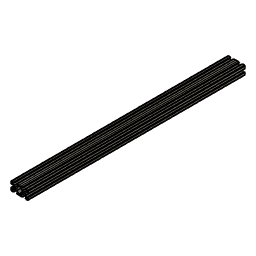
2040-extrusion (Autodesk Fusion 360 design; units mm, degrees)
Autodesk Fusion 360 part; units mm, degrees
sketch "Sketch1" plane through (0, 0, 0) normal (0, 1, 0) x (1, 0, 0)
  line L0 (9, -10) -> (-9, -10)
  line L1 (-10, -9) -> (-10, 9)
  line L2 (-9, 10) -> (9, 10)
  line L3 (10, 9) -> (10, -9)
  line L4 (10, -10) -> (-10, 10) construction
  line L5 (-10, -10) -> (10, 10) construction
  line L6 (4, -4) -> (-4, -4)
  line L7 (-4, -4) -> (-4, 4)
  line L8 (-4, 4) -> (4, 4)
  line L9 (4, 4) -> (4, -4)
  line L10 (4, -4) -> (-4, 4) construction
  line L11 (-4, -4) -> (4, 4) construction
  circle A0 centre (0, 0) radius 2
  line L12 (8.45, -8.45) -> (-8.45, -8.45)
  line L13 (-8.45, -8.45) -> (-8.45, 8.45)
  line L14 (-8.45, 8.45) -> (8.45, 8.45)
  line L15 (8.45, 8.45) -> (8.45, -8.45)
  line L16 (8.45, -8.45) -> (-8.45, 8.45) construction
  line L17 (-8.45, -8.45) -> (8.45, 8.45) construction
  line L18 (-9.452, -10.548) -> (10.548, 9.452) construction
  line L19 (-10.548, -9.452) -> (9.452, 10.548) construction
  line L20 (10.548, -9.452) -> (-9.452, 10.548) construction
  line L21 (9.452, -10.548) -> (-10.548, 9.452) construction
  line L22 (3.1, -10) -> (-3.1, -10) construction
  line L23 (-3.1, -10) -> (-3.1, 10) construction
  line L24 (-3.1, 10) -> (3.1, 10) construction
  line L25 (3.1, 10) -> (3.1, -10) construction
  line L26 (10, -3.1) -> (-10, -3.1) construction
  line L27 (-10, -3.1) -> (-10, 3.1) construction
  line L28 (-10, 3.1) -> (10, 3.1) construction
  line L29 (10, 3.1) -> (10, -3.1) construction
  line L30 (-3.1, -8.45) -> (-3.1, -10)
  line L31 (3.1, -8.45) -> (3.1, -10)
  line L32 (-8.45, -3.1) -> (-10, -3.1)
  line L33 (-8.45, 3.1) -> (-10, 3.1)
  line L34 (8.45, -3.1) -> (10, -3.1)
  line L35 (8.45, 3.1) -> (10, 3.1)
  line L36 (-3.1, 8.45) -> (-3.1, 10)
  line L37 (3.1, 8.45) -> (3.1, 10)
  line L38 (-4, 2.904) -> (-8.45, 7.354)
  line L39 (-2.904, 4) -> (-7.354, 8.45)
  line L40 (2.904, 4) -> (7.354, 8.45)
  line L41 (4, 2.904) -> (8.45, 7.354)
  line L42 (-4, -2.904) -> (-8.45, -7.354)
  line L43 (-2.904, -4) -> (-7.354, -8.45)
  line L44 (2.904, -4) -> (7.354, -8.45)
  line L45 (4, -2.904) -> (8.45, -7.354)
  line L46 (-10, -3.1) -> (-9.55, -3.1)
  line L47 (-9.55, -3.1) -> (-9.55, -3.6)
  line L48 (-9.55, -3.6) -> (-10, -3.6)
  line L49 (-10, -3.6) -> (-10, -3.1)
  line L50 (-10, 3.1) -> (-9.55, 3.1)
  line L51 (-9.55, 3.1) -> (-9.55, 3.6)
  line L52 (-9.55, 3.6) -> (-10, 3.6)
  line L53 (-10, 3.6) -> (-10, 3.1)
  line L54 (-3.1, -10) -> (-3.6, -10)
  line L55 (-3.6, -10) -> (-3.6, -9.55)
  line L56 (-3.6, -9.55) -> (-3.1, -9.55)
  line L57 (-3.1, -9.55) -> (-3.1, -10)
  line L58 (3.1, -10) -> (3.6, -10)
  line L59 (3.6, -10) -> (3.6, -9.55)
  line L60 (3.6, -9.55) -> (3.1, -9.55)
  line L61 (3.1, -9.55) -> (3.1, -10)
  line L62 (10, -3.1) -> (9.55, -3.1)
  line L63 (9.55, -3.1) -> (9.55, -3.6)
  line L64 (9.55, -3.6) -> (10, -3.6)
  line L65 (10, -3.6) -> (10, -3.1)
  line L66 (10, 3.1) -> (9.55, 3.1)
  line L67 (9.55, 3.1) -> (9.55, 3.6)
  line L68 (9.55, 3.6) -> (10, 3.6)
  line L69 (10, 3.6) -> (10, 3.1)
  line L70 (-3.1, 10) -> (-3.6, 10)
  line L71 (-3.6, 10) -> (-3.6, 9.55)
  line L72 (-3.6, 9.55) -> (-3.1, 9.55)
  line L73 (-3.1, 9.55) -> (-3.1, 10)
  line L74 (3.1, 10) -> (3.55, 10)
  line L75 (3.55, 10) -> (3.55, 9.5)
  line L76 (3.55, 9.5) -> (3.1, 9.5)
  line L77 (3.1, 9.5) -> (3.1, 10)
  arc A1 (-10, -9) -> (-9, -10) centre (-9, -9) ccw
  arc A2 (9, -10) -> (10, -9) centre (9, -9) ccw
  arc A3 (10, 9) -> (9, 10) centre (9, 9) ccw
  arc A4 (-9, 10) -> (-10, 9) centre (-9, 9) ccw
  arc A5 (29, -10) -> (30, -9) centre (29, -9) ccw
  line L78 (30, -3.1) -> (10, -3.1) construction
  line L79 (30, 9) -> (30, -9)
  line L80 (24, 4) -> (24, -4)
  line L81 (29.452, -10.548) -> (9.452, 9.452) construction
  line L82 (30, 3.1) -> (29.55, 3.1)
  line L83 (29, -10) -> (11, -10)
  line L84 (16, 4) -> (24, 4)
  line L85 (24, -4) -> (16, 4) construction
  line L86 (28.45, -8.45) -> (11.55, -8.45)
  circle A6 centre (20, 0) radius 2
  line L87 (10, -9) -> (10, 9)
  line L88 (10, -3.1) -> (10, 3.1) construction
  line L89 (16.9, 8.45) -> (16.9, 10)
  arc A7 (11, 10) -> (10, 9) centre (11, 9) ccw
  line L90 (17.096, -4) -> (12.646, -8.45)
  line L91 (16.9, -8.45) -> (16.9, -10)
  line L92 (16.4, -9.55) -> (16.9, -9.55)
  line L93 (10, -3.1) -> (10.45, -3.1)
  line L94 (10, 3.1) -> (10.45, 3.1)
  line L95 (10.45, 3.1) -> (10.45, 3.6)
  arc A8 (10, -9) -> (11, -10) centre (11, -9) ccw
  line L96 (10.45, -3.1) -> (10.45, -3.6)
  line L97 (16.9, -10) -> (16.9, 10) construction
  line L98 (10.45, -3.6) -> (10, -3.6)
  line L99 (29.55, 3.1) -> (29.55, 3.6)
  line L100 (16, -4) -> (16, 4)
  line L101 (23.1, -9.55) -> (23.1, -10)
  line L102 (28.45, -3.1) -> (30, -3.1)
  line L103 (30, -3.6) -> (30, -3.1)
  line L104 (22.904, -4) -> (27.354, -8.45)
  line L105 (22.904, 4) -> (27.354, 8.45)
  line L106 (23.1, 10) -> (23.1, -10) construction
  line L107 (16, -2.904) -> (11.55, -7.354)
  line L108 (16, 2.904) -> (11.55, 7.354)
  line L109 (16.4, 10) -> (16.4, 9.55)
  line L110 (17.096, 4) -> (12.646, 8.45)
  line L111 (10, -3.6) -> (10, -3.1)
  line L112 (16.9, -9.55) -> (16.9, -10)
  line L113 (23.1, 9.5) -> (23.1, 10)
  line L114 (23.6, -10) -> (23.6, -9.55)
  line L115 (10.45, 3.6) -> (10, 3.6)
  line L116 (24, -2.904) -> (28.45, -7.354)
  line L117 (23.55, 10) -> (23.55, 9.5)
  line L118 (10, 3.6) -> (10, 3.1)
  line L119 (11.55, 3.1) -> (10, 3.1)
  line L120 (11.55, -8.45) -> (11.55, 8.45)
  line L121 (23.1, -10) -> (23.6, -10)
  line L122 (11.55, -3.1) -> (10, -3.1)
  line L123 (29.55, -3.6) -> (30, -3.6)
  line L124 (16.4, 9.55) -> (16.9, 9.55)
  line L125 (23.1, 10) -> (23.55, 10)
  line L126 (16.9, 10) -> (16.4, 10)
  line L127 (16.4, -10) -> (16.4, -9.55)
  line L128 (10, 3.1) -> (30, 3.1) construction
  line L129 (24, 2.904) -> (28.45, 7.354)
  line L130 (23.55, 9.5) -> (23.1, 9.5)
  line L131 (23.1, -8.45) -> (23.1, -10)
  line L132 (16.9, 9.55) -> (16.9, 10)
  line L133 (23.1, -10) -> (16.9, -10) construction
  line L134 (30, -3.1) -> (29.55, -3.1)
  line L135 (30.548, -9.452) -> (10.548, 10.548) construction
  line L136 (23.6, -9.55) -> (23.1, -9.55)
  line L137 (29.55, -3.1) -> (29.55, -3.6)
  line L138 (16.9, 10) -> (23.1, 10) construction
  line L139 (30, 3.1) -> (30, -3.1) construction
  line L140 (23.1, 8.45) -> (23.1, 10)
  line L141 (16.9, -10) -> (16.4, -10)
  line L142 (24, -4) -> (16, -4)
  line L143 (16, -4) -> (24, 4) construction
  line L144 (10, -10) -> (30, 10) construction
  arc A9 (30, 9) -> (29, 10) centre (29, 9) ccw
  line L145 (11, 10) -> (29, 10)
  line L146 (28.45, 8.45) -> (28.45, -8.45)
  line L147 (9.452, -9.452) -> (29.452, 10.548) construction
  line L148 (30, 3.6) -> (30, 3.1)
  line L149 (28.45, 3.1) -> (30, 3.1)
  line L150 (11.55, -8.45) -> (28.45, 8.45) construction
  line L151 (11.55, 8.45) -> (28.45, 8.45)
  line L152 (29.55, 3.6) -> (30, 3.6)
  line L153 (30, -10) -> (10, 10) construction
  line L154 (28.45, -8.45) -> (11.55, 8.45) construction
  line L155 (10.548, -10.548) -> (30.548, 9.452) construction
  line L156 (9, -10) -> (11, -10)
  line L157 (9, 10) -> (11, 10)
  line L158 (8.45, -8.45) -> (11.55, -8.45)
  line L159 (8.45, 8.45) -> (11.55, 8.45)
  point P0 (20, 0)
  point P1 (20, 0)
  point P2 (20, 0)
  point P3 (20, 0)
  point P4 (20, 0)
  point P5 (20, 0)
  dimension "d1" = 20
  dimension "d2" = 20
  dimension "d3" = 8
  dimension "d4" = 8
  dimension "d5" = 4
  dimension "d6" = 16.9
  dimension "d7" = 16.9
  dimension "d8" = 0.775
  dimension "d9" = -0.775
  dimension "d10" = 0.775
  dimension "d11" = -0.775
  dimension "d12" = 6.2
  dimension "d13" = 20
  dimension "d14" = 20
  dimension "d15" = 6.2
  dimension "d16" = 1.55
  dimension "d17" = 1.55
  dimension "d18" = 1.55
  dimension "d19" = 1.55
  dimension "d20" = 1.55
  dimension "d21" = 1.55
  dimension "d22" = 1.55
  dimension "d23" = 1.55
  dimension "d24" = 0.45
  dimension "d25" = 0.5
  dimension "d26" = 0.45
  dimension "d27" = 0.5
  dimension "d28" = 0.5
  dimension "d29" = 0.45
  dimension "d30" = 0.5
  dimension "d31" = 0.45
  dimension "d32" = 0.45
  dimension "d33" = 0.5
  dimension "d34" = 0.45
  dimension "d35" = 0.5
  dimension "d36" = 0.5
  dimension "d37" = 0.45
  dimension "d38" = 0.45
  dimension "d39" = 0.5
  dimension "d40" = 1
  dimension "d41" = 1
  dimension "d42" = 1
  dimension "d43" = 1
  dimension "d48" = 0.775
  dimension "d49" = -0.775
  dimension "d50" = 0.775
  dimension "d51" = -0.775
  dimension "d52" = 20
  dimension "d53" = 20
  dimension "d54" = 8
  dimension "d55" = 8
  dimension "d56" = 4
  dimension "d57" = 16.9
  dimension "d58" = 16.9
  dimension "d59" = 6.2
  dimension "d60" = 20
  dimension "d61" = 20
  dimension "d62" = 6.2
  dimension "d63" = 1.55
  dimension "d64" = 1.55
  dimension "d65" = 1.55
  dimension "d66" = 1.55
  dimension "d67" = 1.55
  dimension "d68" = 1.55
  dimension "d69" = 1.55
  dimension "d70" = 1.55
  dimension "d71" = 0.45
  dimension "d72" = 0.5
  dimension "d73" = 0.45
  dimension "d74" = 0.5
  dimension "d75" = 0.5
  dimension "d76" = 0.45
  dimension "d77" = 0.5
  dimension "d78" = 0.45
  dimension "d79" = 0.45
  dimension "d80" = 0.5
  dimension "d81" = 0.45
  dimension "d82" = 0.5
  dimension "d83" = 0.5
  dimension "d84" = 0.45
  dimension "d85" = 0.45
  dimension "d86" = 0.5
  dimension "d87" = 1
  dimension "d88" = 1
  dimension "d89" = 1
  dimension "d90" = 1
  constraint horizontal L0
  constraint perpendicular L0 L1
  constraint parallel L0 L2
  constraint parallel L1 L3
  constraint coincident L4 A0.centre
  constraint coincident L5 A0.centre
  constraint coincident A0.centre origin
  constraint horizontal L6
  constraint perpendicular L6 L7
  constraint parallel L6 L8
  constraint parallel L7 L9
  constraint coincident L10 A0.centre
  constraint coincident L11 A0.centre
  constraint horizontal L12
  constraint perpendicular L12 L13
  constraint parallel L12 L14
  constraint parallel L13 L15
  constraint coincident L16 A0.centre
  constraint coincident L17 A0.centre
  constraint horizontal L22
  constraint perpendicular L22 L23
  constraint parallel L22 L24
  constraint parallel L23 L25
  constraint horizontal L26
  constraint perpendicular L26 L27
  constraint parallel L26 L28
  constraint parallel L27 L29
  constraint vertical L30
  constraint coincident L23 L30.start
  constraint coincident L12 L30.start
  constraint vertical L31
  constraint coincident L12 L31.start
  constraint coincident L25 L31.start
  constraint horizontal L32
  constraint coincident L13 L32.start
  constraint coincident L26 L32.start
  constraint horizontal L33
  constraint coincident L13 L33.start
  constraint coincident L28 L33.start
  constraint horizontal L34
  constraint coincident L15 L34.start
  constraint coincident L26 L34.start
  constraint coincident L28 L35.start
  constraint coincident L15 L35.start
  constraint perpendicular L3 L35
  constraint vertical L36
  constraint coincident L14 L36.start
  constraint coincident L23 L36.start
  constraint vertical L37
  constraint coincident L14 L37.start
  constraint coincident L25 L37.start
  constraint coincident L21 L38.start
  constraint coincident L7 L38.start
  constraint coincident L21 L38.end
  constraint coincident L13 L38.end
  constraint coincident L8 L39.start
  constraint coincident L20 L39.start
  constraint coincident L14 L39.end
  constraint coincident L20 L39.end
  constraint coincident L8 L40.start
  constraint coincident L19 L40.start
  constraint coincident L19 L40.end
  constraint coincident L14 L40.end
  constraint coincident L18 L41.start
  constraint coincident L9 L41.start
  constraint coincident L18 L41.end
  constraint coincident L15 L41.end
  constraint coincident L7 L42.start
  constraint coincident L19 L42.start
  constraint coincident L19 L42.end
  constraint coincident L13 L42.end
  constraint coincident L18 L43.start
  constraint coincident L6 L43.start
  constraint coincident L18 L43.end
  constraint coincident L12 L43.end
  constraint coincident L6 L44.start
  constraint coincident L21 L44.start
  constraint coincident L12 L44.end
  constraint coincident L21 L44.end
  constraint coincident L9 L45.start
  constraint coincident L20 L45.start
  constraint coincident L20 L45.end
  constraint coincident L15 L45.end
  constraint horizontal L46
  constraint vertical L47
  constraint horizontal L48
  constraint vertical L49
  constraint horizontal L50
  constraint vertical L51
  constraint horizontal L52
  constraint vertical L53
  constraint horizontal L54
  constraint vertical L55
  constraint horizontal L56
  constraint vertical L57
  constraint horizontal L58
  constraint vertical L59
  constraint horizontal L60
  constraint vertical L61
  constraint horizontal L62
  constraint vertical L63
  constraint horizontal L64
  constraint vertical L65
  constraint horizontal L66
  constraint vertical L67
  constraint horizontal L68
  constraint vertical L69
  constraint horizontal L70
  constraint vertical L71
  constraint horizontal L72
  constraint vertical L73
  constraint horizontal L74
  constraint vertical L75
  constraint horizontal L76
  constraint vertical L77
  constraint coincident L5.start L0
  constraint coincident L5.start L1
  constraint tangent L0 A1
  constraint tangent L1 A1
  constraint coincident L4.start L0
  constraint coincident L4.start L3
  constraint tangent L0 A2
  constraint tangent L3 A2
  constraint coincident L5.end L3
  constraint coincident L5.end L2
  constraint tangent L3 A3
  constraint tangent L2 A3
  constraint coincident L4.end L2
  constraint coincident L4.end L1
  constraint tangent L2 A4
  constraint tangent L1 A4
  constraint horizontal L83
  constraint perpendicular L83 L87
  constraint parallel L83 L145
  constraint parallel L79 L87
  constraint coincident P5 L153
  constraint coincident P5 L144
  constraint coincident P5 P4
  constraint horizontal L142
  constraint perpendicular L100 L142
  constraint parallel L84 L142
  constraint parallel L80 L100
  constraint coincident P5 L85
  constraint coincident P5 L143
  constraint horizontal L86
  constraint perpendicular L86 L120
  constraint parallel L86 L151
  constraint parallel L120 L146
  constraint coincident P5 L154
  constraint coincident P5 L150
  constraint horizontal L133
  constraint perpendicular L97 L133
  constraint parallel L133 L138
  constraint parallel L97 L106
  constraint horizontal L78
  constraint perpendicular L78 L88
  constraint parallel L78 L128
  constraint parallel L88 L139
  constraint vertical L91
  constraint coincident L91.start L97
  constraint coincident L91.start L86
  constraint vertical L131
  constraint coincident L131.start L86
  constraint coincident L131.start L106
  constraint horizontal L122
  constraint coincident L122.start L120
  constraint coincident L122.start L78
  constraint horizontal L119
  constraint coincident L119.start L120
  constraint coincident L119.start L128
  constraint horizontal L102
  constraint coincident L102.start L146
  constraint coincident L102.start L78
  constraint coincident L149.start L128
  constraint coincident L149.start L146
  constraint perpendicular L79 L149
  constraint vertical L89
  constraint coincident L89.start L151
  constraint coincident L89.start L97
  constraint vertical L140
  constraint coincident L140.start L151
  constraint coincident L140.start L106
  constraint coincident L108.start L81
  constraint coincident L108.start L100
  constraint coincident L108.end L81
  constraint coincident L108.end L120
  constraint coincident L110.start L84
  constraint coincident L110.start L135
  constraint coincident L110.end L151
  constraint coincident L110.end L135
  constraint coincident L105.start L84
  constraint coincident L105.start L147
  constraint coincident L105.end L147
  constraint coincident L105.end L151
  constraint coincident L129.start L155
  constraint coincident L129.start L80
  constraint coincident L129.end L155
  constraint coincident L129.end L146
  constraint coincident L107.start L100
  constraint coincident L107.start L147
  constraint coincident L107.end L147
  constraint coincident L107.end L120
  constraint coincident L90.start L155
  constraint coincident L90.start L142
  constraint coincident L90.end L155
  constraint coincident L90.end L86
  constraint coincident L104.start L142
  constraint coincident L104.start L81
  constraint coincident L104.end L86
  constraint coincident L104.end L81
  constraint coincident L116.start L80
  constraint coincident L116.start L135
  constraint coincident L116.end L135
  constraint coincident L116.end L146
  constraint horizontal L93
  constraint vertical L96
  constraint horizontal L98
  constraint vertical L111
  constraint horizontal L94
  constraint vertical L95
  constraint horizontal L115
  constraint vertical L118
  constraint horizontal L141
  constraint vertical L127
  constraint horizontal L92
  constraint vertical L112
  constraint horizontal L121
  constraint vertical L114
  constraint horizontal L136
  constraint vertical L101
  constraint horizontal L134
  constraint vertical L137
  constraint horizontal L123
  constraint vertical L103
  constraint horizontal L82
  constraint vertical L99
  constraint horizontal L152
  constraint vertical L148
  constraint horizontal L126
  constraint vertical L109
  constraint horizontal L124
  constraint vertical L132
  constraint horizontal L125
  constraint vertical L117
  constraint horizontal L130
  constraint vertical L113
  constraint coincident L4.start L83
  constraint coincident L4.start L87
  constraint tangent L83 A8
  constraint tangent L87 A8
  constraint coincident L153.start L83
  constraint coincident L153.start L79
  constraint tangent A5 L83
  constraint tangent A5 L79
  constraint coincident L144.end L79
  constraint coincident L144.end L145
  constraint tangent L79 A9
  constraint tangent A9 L145
  constraint coincident L5.end L145
  constraint coincident L5.end L87
  constraint tangent A7 L145
  constraint tangent L87 A7
  constraint tangent A8 L156
  measures "d1" distance of L4.end L5.end
  measures "d2" distance of L5.start L4.end
  measures "d3" distance of L7.end L8.end
  measures "d4" distance of L6.end L7.end
  measures "d5" diameter of A0
  measures "d6" distance of L13.end L14.end
  measures "d7" distance of L12.end L13.end
  measures "d12" distance of L23.end L24.end
  measures "d13" distance of L22.end L23.end
  measures "d14" distance of L27.end L28.end
  measures "d15" distance of L26.end L27.end
  measures "d16" distance of L30.start L22.end
  measures "d17" distance of L31.start L22.start
  measures "d18" distance of L32.start L26.end
  measures "d19" distance of L33.start L27.end
  measures "d20" distance of L34.start L26.start
  measures "d21" distance of L35.start L28.end
  measures "d22" distance of L36.start L23.end
  measures "d23" distance of L37.start L24.end
  measures "d24" distance of L26.end L46.end
  measures "d25" distance of L26.end L48.end
  measures "d26" distance of L27.end L50.end
  measures "d27" distance of L27.end L52.end
  measures "d28" distance of L22.end L54.end
  measures "d29" distance of L22.end L56.end
  measures "d30" distance of L22.start L58.end
  measures "d31" distance of L22.start L60.end
  measures "d32" distance of L26.start L62.end
  measures "d33" distance of L26.start L64.end
  measures "d34" distance of L28.end L66.end
  measures "d35" distance of L28.end L68.end
  measures "d36" distance of L23.end L70.end
  measures "d37" distance of L23.end L72.end
  measures "d38" distance of L24.end L74.end
  measures "d39" distance of L24.end L76.end
  measures "d40" radius of A1
  measures "d41" radius of A2
  measures "d42" radius of A3
  measures "d43" radius of A4
  measures "d52" distance of L5.end L144.end
  measures "d53" distance of L4.start L5.end
  measures "d54" distance of L80.start L84.start
  measures "d55" distance of L84.start L100.start
  measures "d56" diameter of A6
  measures "d57" distance of L120.end L146.start
  measures "d58" distance of L120.end L86.end
  measures "d59" distance of L89.end L106.start
  measures "d60" distance of L91.end L89.end
  measures "d61" distance of L82.start L28.end
  measures "d62" distance of L26.start L28.end
  measures "d63" distance of L91.start L91.end
  measures "d64" distance of L101.end L131.start
  measures "d65" distance of L26.start L122.start
  measures "d66" distance of L119.start L28.end
  measures "d67" distance of L102.start L78.start
  measures "d68" distance of L149.start L82.start
  measures "d69" distance of L89.start L89.end
  measures "d70" distance of L140.start L106.start
  measures "d71" distance of L26.start L93.end
  measures "d72" distance of L26.start L64.end
  measures "d73" distance of L94.end L28.end
  measures "d74" distance of L68.end L28.end
  measures "d75" distance of L127.start L91.end
  measures "d76" distance of L92.end L91.end
  measures "d77" distance of L101.end L114.start
  measures "d78" distance of L101.end L101.start
  measures "d79" distance of L134.end L78.start
  measures "d80" distance of L103.start L78.start
  measures "d81" distance of L82.end L82.start
  measures "d82" distance of L148.start L82.start
  measures "d83" distance of L109.start L89.end
  measures "d84" distance of L124.end L89.end
  measures "d85" distance of L117.start L106.start
  measures "d86" distance of L113.start L106.start
  measures "d87" radius of A8
  measures "d88" radius of A5
  measures "d89" radius of A9
  measures "d90" radius of A7
extrude "Extrude2" add sketch "Sketch1" along normal blind 500 contours L0 L3 L12 L31 L59 L60 A2 L87 L158 | A2 A8 L156 | L3 L83 L86 L87 L91 L92 A8 L127 L158 | L6 L9 L12 L15 L44 L45 | L86 L90 L100 L107 L120 L142 | L0 L1 L12 L13 L30 L32 L47 L48 L55 L56 A1 | L6 L7 L8 L9 | L80 L84 L100 L142 | A5 L79 L83 L86 L102 L114 L123 L131 L136 L137 L146 | L6 L7 L12 L13 L42 L43 | L8 L9 L14 L15 L40 L41 | L80 L86 L104 L116 L142 L146 | L84 L100 L108 L110 L120 L151 | L2 L3 L14 L37 L75 L76 A3 L87 L159 | L3 L87 L89 A7 L109 L124 L145 L151 L159 | A3 A7 L157 | L7 L8 L13 L14 L38 L39 | L80 L84 L105 L129 L146 L151 | L1 L2 L13 L14 L33 L36 L51 L52 L71 L72 A4 | L79 L99 L117 L130 L140 A9 L145 L146 L149 L151 L152
equation "d6 = 20 mm - ( ( 1.55 * 2 ) * 1 mm )"
equation "d7 = 20 mm - ( ( 1.55 * 2 ) * 1 mm )"
equation "d8 = ( 1.55 / 2 ) * 1 mm"
equation "d9 = ( -1.55 / 2 ) * 1 mm"
equation "d10 = ( 1.55 / 2 ) * 1 mm"
equation "d11 = ( -1.55 / 2 ) * 1 mm"
equation "d48 = ( 1.55 / 2 ) * 1 mm"
equation "d49 = ( -1.55 / 2 ) * 1 mm"
equation "d50 = ( 1.55 / 2 ) * 1 mm"
equation "d51 = ( -1.55 / 2 ) * 1 mm"
equation "d57 = 20 mm - ( ( 1.55 * 2 ) * 1 mm )"
equation "d58 = 20 mm - ( ( 1.55 * 2 ) * 1 mm )"
named bodies: "2040-extrusion"
